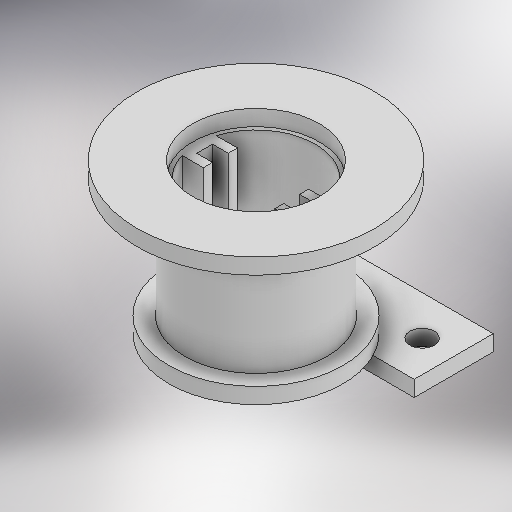
# Autodesk Inventor part: tmrEXCI
Saved by Autodesk Inventor 2025.2 (Build 292293000, 293)
## iProperties
Created: 2025-08-15
Part Number: tmrEXCI
Material: 一般
Document SubType Name: Modeling
Designer: 123
Density: 1 g/cm^3
Appearance: 預設
Author: 123
Autodesk Inventor part; units mm, degrees
ref_plane "YZ Plane" through (0, 0, 0) normal (1, 0, 0) x (0, 1, 0)
ref_plane "XZ Plane" through (0, 0, 0) normal (0, 1, 0) x (-1, 0, 0)
ref_plane "XY Plane" through (0, 0, 0) normal (0, 0, 1) x (1, 0, 0)
sketch "草圖1" plane through (0, 0, 0) normal (0, 1, 0) x (-1, 0, 0)
  circle A0 centre (0, 0) radius 7.5
  circle A1 centre (0, 0) radius 9
  line L0 (7.5, 2.1585) -> (4.5, 2.1585)
  line L1 (4.5, 2.1585) -> (4.5, -2.1585)
  line L2 (4.5, -2.1585) -> (7.5, -2.1585)
  line L3 (7.5, -2.1585) -> (7.5, 2.1585)
  line L4 (7, 1) -> (4.5, 1)
  line L5 (4.5, 1) -> (4.5, -1)
  line L6 (4.5, -1) -> (7, -1)
  line L7 (7, -1) -> (7, 1)
  line L8 (0, 5.058) -> (0, -5.7034)
  line L9 (-7.5, 2.1585) -> (-4.5, 2.1585)
  line L10 (-4.5, 2.1585) -> (-4.5, -2.1585)
  line L11 (-4.5, -2.1585) -> (-7.5, -2.1585)
  line L12 (-7.5, -2.1585) -> (-7.5, 2.1585)
  line L13 (-7, 1) -> (-4.5, 1)
  line L14 (-4.5, -1) -> (-7, -1)
  line L15 (-7, -1) -> (-7, 1)
  point P0 (5.75, -1)
  point P1 (7.5, 0)
  point P2 (-7.1827, 2.1585)
  point P3 (7.1827, 2.1585)
  point P4 (4.5, 1)
  point P5 (7.1827, -2.1585)
  point P6 (-7.1827, -2.1585)
  point P7 (-4.5, 1)
  dimension "d0" = 15
  dimension "d1" = 18
  dimension "d2" = 2
  dimension "d3" = 1
  dimension "d4" = 0
  dimension "d5" = 2.5
  dimension "d28" = 3
  constraints: 32 end point, 8 symmetric about line, 4 parallel, 2 centre point, 2 coincident, 2 horizontal, 2 midpoint, 2 perpendicular, 2 point on line, 1 tangent, 1 vertical
  measures "d0" diameter of A0
  measures "d1" diameter of A1
  measures "d2" distance from line of point (5.75, -1) L4
  measures "d3" vertical distance of point (0, 0) point (5.75, -1)
  measures "d4" vertical distance of point (0, 0) point (7.5, 0)
  measures "d5" distance between parallel lines of L1 L7
  measures "d28" distance of L10.end L12.start
extrude "擠出1" add sketch "草圖1" along normal blind 15 contours A0 L2 L1 L6 L7 L4 L0 | L3 L2 A0 | A0 L0 L3 | L9 L10 L13 L15 L14 L11 A0 | A0 L12 L9 | L11 L12 A0 | A1
sketch "草圖2" plane through (0, 15, 0) normal (0, 1, 0) x (1, 0, 0)
  circle A0 centre (0, 0) radius 15
  circle A1 centre (0, 0) radius 8
  dimension "d8" = 30
  dimension "d23" = 16
  constraints: 2 centre point, 2 coincident
  measures "d8" diameter of A0
  measures "d23" diameter of A1
extrude "擠出2" add sketch "草圖2" along normal blind 2
sketch "草圖3" plane through (0, 0, 0) normal (0, -1, 0) x (1, 0, 0)
  circle A0 centre (0, 0) radius 11
  line L0 (-4.5, -2.1585) -> (-7.1827, -2.1585) projected
  circle A1 centre (0, 0) radius 7.5
  constraints: 2 coincident, 1 centre point, 3 other
extrude "擠出3" add sketch "草圖3" along normal blind 2
sketch "草圖4" plane through (0, -2, 0) normal (0, -1, 0) x (1, 0, 0)
  line L0 (-15, -15) -> (15, -15)
  line L1 (15, -15) -> (15, -5)
  line L2 (-15, -5) -> (-15, -15)
  circle A0 centre (0, 0) radius 7.5 projected
  circle A1 centre (11, -10) radius 1.55
  circle A2 centre (-11, -10) radius 1.55
  line L3 (-15, -5) -> (15, -5)
  point P0 (0, -15)
  point P1 (-15, -10)
  point P2 (15, -10)
  dimension "d13" = 30
  dimension "d14" = 0
  dimension "d15" = 10
  dimension "d16" = 3.1
  dimension "d17" = 3.1
  dimension "d18" = 11
  dimension "d19" = 11
  dimension "d22" = 5
  constraints: 8 end point, 3 midpoint, 2 centre point, 2 horizontal, 2 horizontal alignment, 1 parallel, 1 perpendicular
  measures "d13" distance of L0.start L0.end
  measures "d14" horizontal distance of point (0, 0) point (0, -15)
  measures "d15" distance of L2.start L0.start
  measures "d16" diameter of A2
  measures "d17" diameter of A1
  measures "d18" horizontal distance of point (0, 0) A2.centre
  measures "d19" horizontal distance of point (0, 0) A1.centre
  measures "d22" distance from line of point (0, 0) L3
extrude "擠出4" add sketch "草圖4" along normal blind 2 contours L2 L3 A0 L1 L0 | L3 A0 picked at (1.4132, -5.3956)
sketch "草圖5" plane through (0, 0, 0) normal (0, -1, 0) x (1, 0, 0)
  line L0 (7, -1) -> (7, 1) projected
  line L1 (7, 1) -> (4.5, 1) projected
  line L2 (7, -1) -> (6.5, -1)
  line L3 (6.5, -1) -> (6.5, 1)
  line L4 (6.5, 1) -> (7, 1)
  line L5 (7, 1) -> (7, -1)
  line L6 (-7, -1) -> (-4.5, -1) projected
  line L7 (-7, 1) -> (-7, -1) projected
  line L8 (-6.5, -1) -> (-7, -1)
  line L9 (-7, -1) -> (-7, 1)
  line L10 (-7, 1) -> (-6.5, 1)
  line L11 (-6.5, 1) -> (-6.5, -1)
  point P0 (0, 0)
  dimension "d24" = 0.5
  dimension "d25" = 0.5
  constraints: 16 end point, 4 parallel, 2 horizontal, 2 perpendicular, 2 point on line
  measures "d24" distance of L0.start L2.end
  measures "d25" distance of L6.start L8.start
extrude "擠出5" add sketch "草圖5" against normal blind 15
